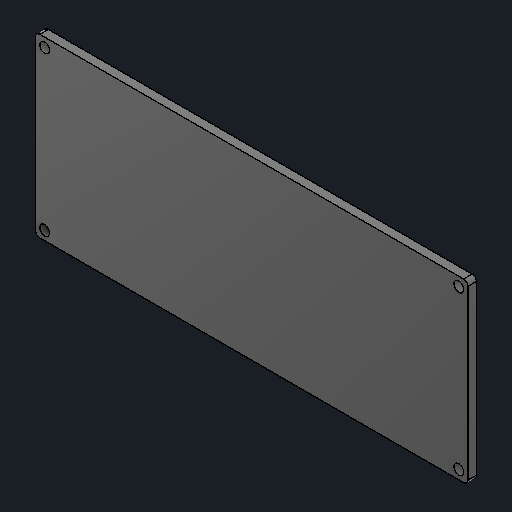
# Autodesk Inventor part: Junction Box Modbay Cover
Saved by Autodesk Inventor 2026.2 (Build 302298000, 298)
## iProperties
Created: 2026-08-25
Part Number: Junction Box Modbay Cover
Material: ABS Plastic
Document SubType Name: Modeling
Designer: JoshuaEah
Density: 1.06 g/cm^3
Appearance: Smooth - Black
Author: JoshuaEah
Autodesk Inventor part; units mm, degrees
ref_plane "YZ Plane" through (0, 0, 0) normal (1, 0, 0) x (0, 1, 0)
ref_plane "XZ Plane" through (0, 0, 0) normal (0, 1, 0) x (-1, 0, 0)
ref_plane "XY Plane" through (0, 0, 0) normal (0, 0, 1) x (1, 0, 0)
sketch "Main Profile" plane through (0, 0, 0) normal (0, 0, 1) x (1, 0, 0)
  line L0 (0, 0) -> (152, 0)
  line L1 (152, 0) -> (152, 62)
  line L2 (152, 62) -> (0, 62)
  line L3 (0, 62) -> (0, 0)
  line L4 (0, 31) -> (152, 31)
  line L5 (76, 62) -> (76, 0)
  point P0 (3.175, 58.825)
  point P1 (148.825, 58.825)
  point P2 (3.175, 3.175)
  point P3 (148.825, 3.175)
  dimension "d0" = 152
  dimension "d1" = 62
  dimension "d2" = 3.175
  dimension "d3" = 3.175
  constraints: 12 end point, 4 midpoint, 3 symmetric about line, 2 parallel, 1 coincident, 1 horizontal, 1 perpendicular
  measures "d0" distance of L1.end L2.end
  measures "d1" distance of L0.end L1.end
  measures "d2" distance from line of L3 point (3.175, 58.825)
  measures "d3" distance from line of L2 point (3.175, 58.825)
extrude "Panel" add sketch "Main Profile" against normal blind 3
hole "Mounting Hole" at (3.175, 58.825, 0) direction (0, 0, -1) diameter 3.4036 end through all start extended yes clearance for "Socket Head Cap Screw" size "M3" standard "Ansi Metric M Profile"
pattern_sketch "Mounting Holes" of "Mounting Hole" from (3.175, 58.825, 0) copies at (148.825, 58.825, 0) at (3.175, 3.175, 0) at (148.825, 3.175, 0)
fillet "Corner Fillets" radius 1.5 4 edges at (0, 62, -1.5) (0, 0, -1.5) (152, 0, -1.5) (152, 62, -1.5)
equation "\"d3\" = d2"
body "Solid1"
